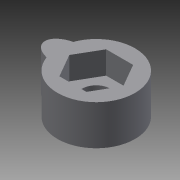
# Autodesk Inventor part: cam4.0
Saved by Autodesk Inventor 2014 (Build 180170000, 170)
## iProperties
Created: 2014-02-14
Part Number: cam4.0
Material: Generic
Document SubType Name: Modeling
Designer: stephen
Density: 1 g/cm^3
Appearance: Default
Author: stephen
Autodesk Inventor part; units mm, degrees
ref_plane "YZ Plane" through (0, 0, 0) normal (1, 0, 0) x (0, 1, 0)
ref_plane "XZ Plane" through (0, 0, 0) normal (0, 1, 0) x (-1, 0, 0)
ref_plane "XY Plane" through (0, 0, 0) normal (0, 0, 1) x (1, 0, 0)
sketch "Sketch1" plane through (0, 0, 0) normal (0, 0, 1) x (1, 0, 0)
  line L0 (-2.5, 0) -> (-9, 0)
  ellipse E0 centre (-4.792, 0) end of major axis (-9, 0) minor radius 2.5316 (-6.3785, 2.3447) -> (-6.3785, -2.3447) ccw
  arc A0 (-6.3785, -2.3447) -> (-6.3785, 2.3447) centre (0, 0) ccw
  line L1 (-6.3785, 2.3447) -> (-6.225, 2.482)
  circle A1 centre (0, 0) radius 2.5
  dimension "d2" = 6.5
  dimension "d4" = 5
  constraints: 4 end point, 2 centre point, 2 point on circle, 1 coincident, 1 horizontal, 5 other
  measures "d2" distance of L0.start L0.end
  measures "d4" diameter of A1
extrude "Extrusion1" add sketch "Sketch1" along normal blind 7
sketch "Sketch2" plane through (0, 0, 7) normal (0, 0, 1) x (1, 0, 0)
  circle A0 centre (0, 0) radius 2.5 projected
  arc A1 (-6.3785, -2.3447) -> (-6.3785, 2.3447) centre (0, 0) ccw projected
  line L0 (4.7343, 0) -> (2.3671, -4.1)
  line L1 (2.3671, -4.1) -> (-2.3671, -4.1)
  line L2 (-2.3671, -4.1) -> (-4.7343, 0)
  line L3 (-4.7343, 0) -> (-2.3671, 4.1)
  line L4 (-2.3671, 4.1) -> (2.3671, 4.1)
  line L5 (2.3671, 4.1) -> (4.7343, 0)
  dimension "d7" = 8.2
  constraints: 12 end point, 1 coincident, 13 other
  measures "d7" distance between parallel lines of L1 L4
extrude "Extrusion2" cut sketch "Sketch2" against normal blind 4
body "Solid1"
